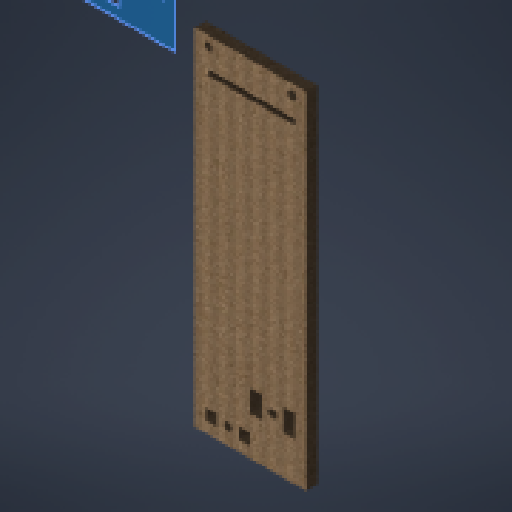
# Autodesk Inventor part: Door_V2
Saved by Autodesk Inventor 2024.1 (Build 281209000, 209)
## iProperties
Created: 2023-05-15
Part Number: Door_V2
Material: MDF Medium Density Fiberboard
Document SubType Name: Modeling
Designer: jaege
Density: 0.8 g/cm^3
Appearance: Cardboard - Corrugated
Author: jaege
Autodesk Inventor part; units mm, degrees
ref_plane "YZ Plane" through (0, 0, 0) normal (1, 0, 0) x (0, 1, 0)
ref_plane "XZ Plane" through (0, 0, 0) normal (0, 1, 0) x (-1, 0, 0)
ref_plane "XY Plane" through (0, 0, 0) normal (0, 0, 1) x (1, 0, 0)
sketch "Sketch1" plane through (0, 0, 0) normal (0, 1, 0) x (-1, 0, 0)
  line L0 (20, 2) -> (-20, 2)
  line L1 (-20, 2) -> (-20, -2)
  line L2 (-20, -2) -> (20, -2)
  line L3 (20, -2) -> (20, 2)
  line L4 (20, 2) -> (-20, -2) construction
  line L5 (-20, 2) -> (20, -2) construction
  point P0 (0, 0)
  dimension "d0" = 40
  dimension "d1" = 4
  constraints: 12 end point, 2 midpoint, 2 parallel, 1 horizontal, 1 perpendicular
  measures "d0" distance of L1.end L2.end
  measures "d1" distance of L0.end L1.end
extrude "Extrusion1" add sketch "Sketch1" along normal blind 84
sketch "Sketch2" plane through (0, 84, 0) normal (0, 1, 0) x (1, 0, 0)
  line L0 (20, 2) -> (-20, 2) projected
  line L1 (20, -2) -> (20, 2) projected
  line L2 (20, 2) -> (-20, 2) projected
  line L3 (-20, 2) -> (-20, -2) projected
  line L4 (-20, -2) -> (20, -2) projected
  point P0 (0, 0)
extrude "Extrusion2" add sketch "Sketch2" along normal blind 14
sketch "Sketch3" plane through (-20, 0, 2) normal (0, 0, 1) x (1, 0, 0)
  line L0 (0, 98) -> (40, 98) projected
  line L1 (20, 98) -> (20, 0)
  line L2 (40, 0) -> (0, 0) projected
  point P0 (5, 94.45)
  point P1 (35, 94.45)
  dimension "d6" = 3.55
  dimension "d7" = 30
  constraints: 2 end point, 1 horizontal alignment, 1 midpoint, 1 perpendicular, 1 symmetric about line
  measures "d6" distance from line of L0 point (5, 94.45)
  measures "d7" distance of point (35, 94.45) point (5, 94.45)
hole "Hole1" at (-15, 94.45, 2) at (15, 94.45, 2) direction (0, 0, -1) diameter 3.1 depth 4
sketch "Sketch4" plane through (-20, 0, 2) normal (0, 0, 1) x (1, 0, 0)
  line L0 (4, 85.45) -> (36, 85.45)
  circle A0 centre (5, 94.45) radius 1.55 projected
  circle A1 centre (35, 94.45) radius 1.55 projected
  line L1 (0, 0) -> (40, 0) projected
  line L2 (40, 0) -> (40, 98) projected
  line L3 (0, 98) -> (40, 98) projected
  line L4 (0, 0) -> (0, 98) projected
  line L5 (40, 0) -> (40, 98) projected
  line L6 (4, 85.45) -> (36, 85.45)
  line L7 (36, 85.45) -> (36, 87.4)
  line L8 (36, 87.4) -> (4, 87.4)
  line L9 (4, 87.4) -> (4, 85.45)
  line L10 (0, 98) -> (40, 98) projected
  point P0 (20, 0)
  point P1 (20, 98)
  point P2 (20, 85.45)
  point P3 (0, 87.4)
  point P4 (40, 87.4)
  point P5 (37.1403, 85.45)
  point P6 (20, 98)
  dimension "d16" = 1.95
  dimension "d33" = 12.55
  dimension "d44" = 4
  constraints: 10 end point, 3 midpoint, 2 horizontal, 2 parallel, 1 perpendicular, 1 vertical alignment, 1 other
  measures "d16" distance between parallel lines of L0 L8
  measures "d33" distance between parallel lines of L3 L0
  measures "d44" distance between parallel lines of L2 L7
extrude "IndicatorBar" cut sketch "Sketch4" against normal blind 1 contours L9 L8 L7 L0
sketch "Sketch6" plane through (-20, 0, 2) normal (0, 0, 1) x (1, 0, 0)
  line L0 (40, 0) -> (0, 0) projected
  line L1 (0, 0) -> (40, 0)
  line L2 (40, 0) -> (40, -26)
  line L3 (40, -26) -> (0, -26)
  line L4 (0, -26) -> (0, 0)
  line L5 (40, 0) -> (40, 98) projected
  line L6 (20, -4) -> (24, -4)
  line L7 (24, -4) -> (24, -8)
  line L8 (24, -8) -> (20, -8)
  line L9 (20, -8) -> (20, -4)
  line L10 (32, -8) -> (36, -8)
  line L11 (36, -8) -> (36, -4)
  line L12 (36, -4) -> (32, -4)
  line L13 (32, -4) -> (32, -8)
  line L14 (4, -18) -> (8, -18)
  line L15 (8, -18) -> (8, -22)
  line L16 (8, -22) -> (4, -22)
  line L17 (4, -22) -> (4, -18)
  line L18 (16, -22) -> (20, -22)
  line L19 (20, -22) -> (20, -18)
  line L20 (20, -18) -> (16, -18)
  line L21 (16, -18) -> (16, -22)
  circle A0 centre (12, -20) radius 1.5
  line L22 (8, -18) -> (16, -22) construction
  line L23 (20, -8) -> (24, -8)
  line L24 (24, -8) -> (24, -12)
  line L25 (24, -12) -> (20, -12)
  line L26 (20, -12) -> (20, -8)
  line L27 (32, -8) -> (36, -8)
  line L28 (36, -8) -> (36, -12)
  line L29 (36, -12) -> (32, -12)
  line L30 (32, -12) -> (32, -8)
  line L31 (24, -4) -> (32, -12) construction
  circle A1 centre (28, -8) radius 1.5
  point P0 (20, 0)
  point P1 (40, 85.45)
  point P2 (36, -6)
  point P3 (8, -20)
  point P4 (6, -22)
  point P5 (4, -20)
  point P6 (20, -4)
  point P7 (20, -12)
  point P8 (18, -18)
  point P9 (32, -10)
  dimension "d24" = 4
  dimension "d25" = 4
  dimension "d26" = 4
  dimension "d28" = 4
  dimension "d29" = 4
  dimension "d30" = 4
  dimension "d34" = 4
  dimension "d35" = 4
  dimension "d36" = 3
  dimension "d37" = 10
  dimension "d38" = 4
  dimension "d39" = 4
  dimension "d40" = 4
  dimension "d41" = 4
  dimension "d43" = 3
  constraints: 60 end point, 14 parallel, 8 midpoint, 7 horizontal, 7 perpendicular, 4 point on line, 3 collinear, 2 centre point, 1 coincident, 1 vertical alignment, 2 other
  measures "d24" distance from line of L0 L11.end
  measures "d25" distance from line of L2 point (36, -6)
  measures "d26" distance of L14.start L14.end
  measures "d28" distance of L16.end L14.start
  measures "d29" distance from line of L3 point (6, -22)
  measures "d30" distance from line of L4 point (4, -20)
  measures "d34" distance of L10.end L11.end
  measures "d35" distance of L11.end L12.end
  measures "d36" diameter of A0
  measures "d37" distance from line of point (18, -18) L8
  measures "d38" distance of L23.end L24.end
  measures "d39" distance of L28.end L29.end
  measures "d40" distance of L27.end L28.end
  measures "d41" distance of L24.end L25.end
  measures "d43" diameter of A1
extrude "UnderCar" add sketch "Sketch6" against normal blind 4
body "Solid1"
